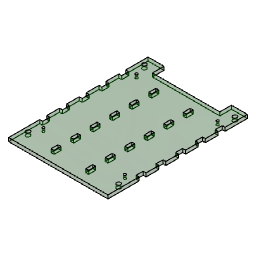
Support_batteries_PCB_KOSMOS3-0 (Autodesk Fusion 360 design; units mm, degrees)
Autodesk Fusion 360 part; units mm, degrees
sketch "Esquisse1" plane through (0, 0, 0) normal (0, 0, 1) x (1, 0, 0)
  line L0 (0, 0) -> (-85.47, 0)
  line L1 (-85.47, 0) -> (-85.47, 120)
  line L2 (0, 120) -> (0, 0)
  circle A0 centre (-81.67, 13) radius 1.75
  circle A1 centre (-3.8, 13) radius 1.75
  circle A2 centre (-81.67, 113) radius 1.75
  circle A3 centre (-3.8, 113) radius 1.75
  line L3 (-71.735, 120) -> (-71.735, 110)
  line L4 (-71.735, 110) -> (-13.735, 110)
  line L5 (-13.735, 110) -> (-13.735, 120)
  line L6 (-85.47, 120) -> (-71.735, 120)
  line L7 (-13.735, 120) -> (0, 120)
  dimension "d1" = 85.47
  dimension "d3" = 77.87
  dimension "d5" = 3.8
  dimension "d6" = 3.5
  dimension "d7" = 3.5
  dimension "d8" = 13
  dimension "d9" = 3.5
  dimension "d10" = 3.5
  dimension "d13" = 13
  dimension "d14" = 3.8
  dimension "d15" = 77.87
  dimension "d16" = 58
  dimension "d17" = 10
  dimension "d18" = 13.735
  dimension "d21" = 120
  dimension "d22" = 7
  dimension "d24" = 7
  constraint horizontal L0
  constraint vertical L1
  constraint vertical L2
  constraint coincident L0.start L2.end
  constraint perpendicular L3 L4
  constraint perpendicular L3 L6
  constraint perpendicular L2 L7
  constraint equal L1 L2
  measures "d1" distance of L0.start L0.end
  measures "d3" distance of A0.centre A1.centre
  measures "d5" distance of L1 A0.centre
  measures "d6" diameter of A1
  measures "d7" diameter of A0
  measures "d8" distance of L0 A0.centre
  measures "d9" diameter of A3
  measures "d10" diameter of A2
  measures "d13" distance of L0 A1.centre
  measures "d14" distance of L1 A2.centre
  measures "d15" distance of A2.centre A3.centre
  measures "d16" distance of L3.end L4.end
  measures "d17" distance of L4.end L5.end
  measures "d18" distance of L2 L5
  measures "d21" distance of L0.start L2.start
  measures "d22" distance of A3.centre L7
  measures "d24" distance of A2.centre L6
extrude "Extrusion1" add sketch "Esquisse1" along normal blind 3
sketch "Esquisse2" plane through (0, 0, 3) normal (0, 0, 1) x (-1, 0, 0)
  circle A0 centre (3.8, -113) radius 1.75
  circle A1 centre (81.67, -113) radius 1.75
  circle A2 centre (3.8, -13) radius 1.75
  circle A3 centre (81.67, -13) radius 1.75
  line L0 (13.735, -120) -> (13.735, -110)
  line L1 (13.735, -110) -> (71.735, -110)
  line L2 (71.735, -110) -> (71.735, -120)
  line L3 (71.735, -120) -> (85.47, -120)
  line L4 (85.47, -120) -> (85.47, 0)
  line L5 (85.47, 0) -> (0, 0)
  line L6 (0, 0) -> (0, -120)
  line L7 (0, -120) -> (13.735, -120)
  line L8 (58.87, -10) -> (56.37, -10)
  line L9 (56.37, -10) -> (56.37, -16)
  line L10 (56.37, -16) -> (58.87, -16)
  line L11 (58.87, -16) -> (58.87, -10)
  line L12 (56.37, -26.8) -> (56.37, -32.8)
  line L13 (56.37, -32.8) -> (58.87, -32.8)
  line L14 (58.87, -26.8) -> (56.37, -26.8)
  line L15 (58.87, -32.8) -> (58.87, -26.8)
  line L16 (56.37, -43.6) -> (56.37, -49.6)
  line L17 (56.37, -49.6) -> (58.87, -49.6)
  line L18 (58.87, -43.6) -> (56.37, -43.6)
  line L19 (58.87, -49.6) -> (58.87, -43.6)
  line L20 (56.37, -60.4) -> (56.37, -66.4)
  line L21 (56.37, -66.4) -> (58.87, -66.4)
  line L22 (58.87, -60.4) -> (56.37, -60.4)
  line L23 (58.87, -66.4) -> (58.87, -60.4)
  line L24 (56.37, -77.2) -> (56.37, -83.2)
  line L25 (56.37, -83.2) -> (58.87, -83.2)
  line L26 (58.87, -77.2) -> (56.37, -77.2)
  line L27 (58.87, -83.2) -> (58.87, -77.2)
  line L28 (56.37, -94) -> (56.37, -100)
  line L29 (56.37, -100) -> (58.87, -100)
  line L30 (58.87, -94) -> (56.37, -94)
  line L31 (58.87, -100) -> (58.87, -94)
  line L32 (42.735, 23.8439) -> (42.735, -200) construction
  line L33 (42.735, 7.0439) -> (42.735, -216.8) construction
  line L34 (29.1, -83.2) -> (26.6, -83.2)
  line L35 (26.6, -10) -> (29.1, -10)
  line L36 (29.1, -16) -> (26.6, -16)
  line L37 (29.1, -66.4) -> (26.6, -66.4)
  line L38 (29.1, -10) -> (29.1, -16)
  line L39 (29.1, -49.6) -> (26.6, -49.6)
  line L40 (26.6, -77.2) -> (29.1, -77.2)
  line L41 (26.6, -94) -> (29.1, -94)
  line L42 (26.6, -49.6) -> (26.6, -43.6)
  line L43 (29.1, -77.2) -> (29.1, -83.2)
  line L44 (29.1, -94) -> (29.1, -100)
  line L45 (26.6, -83.2) -> (26.6, -77.2)
  line L46 (29.1, -32.8) -> (26.6, -32.8)
  line L47 (29.1, -26.8) -> (29.1, -32.8)
  line L48 (29.1, -60.4) -> (29.1, -66.4)
  line L49 (26.6, -26.8) -> (29.1, -26.8)
  line L50 (26.6, -32.8) -> (26.6, -26.8)
  line L51 (26.6, -60.4) -> (29.1, -60.4)
  line L52 (26.6, -16) -> (26.6, -10)
  line L53 (29.1, -43.6) -> (29.1, -49.6)
  line L54 (29.1, -100) -> (26.6, -100)
  line L55 (26.6, -100) -> (26.6, -94)
  line L56 (26.6, -43.6) -> (29.1, -43.6)
  line L57 (26.6, -66.4) -> (26.6, -60.4)
  line L58 (85.47, -26.8) -> (82.97, -26.8)
  line L59 (82.97, -26.8) -> (82.97, -32.8)
  line L60 (82.97, -32.8) -> (85.47, -32.8)
  line L61 (85.47, -32.8) -> (85.47, -26.8)
  line L62 (82.97, -43.8) -> (82.97, -49.8)
  line L63 (82.97, -49.8) -> (85.47, -49.8)
  line L64 (85.47, -49.8) -> (85.47, -43.8)
  line L65 (85.47, -43.8) -> (82.97, -43.8)
  line L66 (82.97, -60.8) -> (82.97, -66.8)
  line L67 (82.97, -66.8) -> (85.47, -66.8)
  line L68 (85.47, -66.8) -> (85.47, -60.8)
  line L69 (85.47, -60.8) -> (82.97, -60.8)
  line L70 (82.97, -77.8) -> (82.97, -83.8)
  line L71 (82.97, -83.8) -> (85.47, -83.8)
  line L72 (85.47, -83.8) -> (85.47, -77.8)
  line L73 (85.47, -77.8) -> (82.97, -77.8)
  line L74 (82.97, -94.8) -> (82.97, -100.8)
  line L75 (82.97, -100.8) -> (85.47, -100.8)
  line L76 (85.47, -100.8) -> (85.47, -94.8)
  line L77 (85.47, -94.8) -> (82.97, -94.8)
  line L78 (2.5, -43.8) -> (2.5, -49.8)
  line L79 (2.5, -100.8) -> (0, -100.8)
  line L80 (0, -49.8) -> (0, -43.8)
  line L81 (2.5, -77.8) -> (2.5, -83.8)
  line L82 (0, -83.8) -> (0, -77.8)
  line L83 (0, -77.8) -> (2.5, -77.8)
  line L84 (0, -26.8) -> (2.5, -26.8)
  line L85 (0, -32.8) -> (0, -26.8)
  line L86 (2.5, -49.8) -> (0, -49.8)
  line L87 (0, -100.8) -> (0, -94.8)
  line L88 (0, -60.8) -> (2.5, -60.8)
  line L89 (2.5, -32.8) -> (0, -32.8)
  line L90 (2.5, -83.8) -> (0, -83.8)
  line L91 (2.5, -94.8) -> (2.5, -100.8)
  line L92 (2.5, -66.8) -> (0, -66.8)
  line L93 (2.5, -26.8) -> (2.5, -32.8)
  line L94 (2.5, -60.8) -> (2.5, -66.8)
  line L95 (0, -43.8) -> (2.5, -43.8)
  line L96 (0, -66.8) -> (0, -60.8)
  line L97 (0, -94.8) -> (2.5, -94.8)
  dimension "d25" = 2.5
  dimension "d26" = 6
  dimension "d27" = 26.6
  dimension "d31" = -20
  dimension "d32" = -84
  dimension "d35" = 85.47
  dimension "d37" = 42.735
  dimension "d42" = 2.5
  dimension "d43" = 6
  dimension "d44" = 26.8
  dimension "d45" = 26.8
  dimension "d48" = 0
  dimension "d49" = -68
  constraint horizontal L8
  constraint vertical L9
  constraint horizontal L10
  constraint vertical L11
  constraint perpendicular L1 L32
  constraint horizontal L58
  constraint vertical L59
  constraint horizontal L60
  constraint vertical L61
  constraint coincident L4 L58.start
  measures "d25" distance of L8.start L8.end
  measures "d26" distance of L8.start L10.end
  measures "d27" distance of L4 L11
  measures "d35" distance of L4.end L5.end
  measures "d37" distance of L4 L32
  measures "d42" distance of L58.start L58.end
  measures "d43" distance of L58.end L59.end
  measures "d44" distance of L5 L14
  measures "d45" distance of L5 L58
extrude "Extrusion2" cut sketch "Esquisse2" against normal blind 3 contours L6 L79 L87 L91 L97 | L6 L81 L82 L83 L90 | L4 L74 L75 L76 L77 | L6 L88 L92 L94 L96 | L4 L70 L71 L72 L73 | L6 L78 L80 L86 L95 | L4 L66 L67 L68 L69 | L6 L84 L85 L89 L93 | L4 L62 L63 L64 L65 | L4 L58 L59 L60 L61 | L8 L9 L10 L11 | L12 L13 L14 L15 | L16 L17 L18 L19 | L20 L21 L22 L23 | L24 L25 L26 L27 | L28 L29 L30 L31 | L34 L40 L43 L45 | L35 L36 L38 L52 | L37 L48 L51 L57 | L39 L42 L53 L56 | L41 L44 L54 L55 | L46 L47 L49 L50
sketch "Esquisse3" plane through (0, 0, 3) normal (0, 0, 1) x (-1, 0, 0)
  line L0 (2.5, -32.8) -> (0, -32.8)
  line L1 (0, -32.8) -> (0, -43.8)
  line L2 (0, -43.8) -> (2.5, -43.8)
  line L3 (2.5, -43.8) -> (2.5, -49.8)
  line L4 (2.5, -49.8) -> (0, -49.8)
  line L5 (0, -49.8) -> (0, -60.8)
  line L6 (0, -60.8) -> (2.5, -60.8)
  line L7 (2.5, -60.8) -> (2.5, -66.8)
  line L8 (2.5, -66.8) -> (0, -66.8)
  line L9 (0, -66.8) -> (0, -77.8)
  line L10 (0, -77.8) -> (2.5, -77.8)
  line L11 (2.5, -77.8) -> (2.5, -83.8)
  line L12 (2.5, -83.8) -> (0, -83.8)
  line L13 (0, -83.8) -> (0, -94.8)
  line L14 (0, -94.8) -> (2.5, -94.8)
  line L15 (2.5, -94.8) -> (2.5, -100.8)
  line L16 (2.5, -100.8) -> (0, -100.8)
  line L17 (0, -100.8) -> (0, -120)
  line L18 (0, -120) -> (13.735, -120)
  line L19 (13.735, -120) -> (13.735, -110)
  line L20 (13.735, -110) -> (71.735, -110)
  line L21 (71.735, -110) -> (71.735, -120)
  line L22 (71.735, -120) -> (85.47, -120)
  line L23 (85.47, -120) -> (85.47, -100.8)
  line L24 (85.47, -100.8) -> (82.97, -100.8)
  line L25 (82.97, -100.8) -> (82.97, -94.8)
  line L26 (82.97, -94.8) -> (85.47, -94.8)
  line L27 (85.47, -94.8) -> (85.47, -83.8)
  line L28 (85.47, -83.8) -> (82.97, -83.8)
  line L29 (82.97, -83.8) -> (82.97, -77.8)
  line L30 (82.97, -77.8) -> (85.47, -77.8)
  line L31 (85.47, -77.8) -> (85.47, -66.8)
  line L32 (85.47, -66.8) -> (82.97, -66.8)
  line L33 (82.97, -66.8) -> (82.97, -60.8)
  line L34 (82.97, -60.8) -> (85.47, -60.8)
  line L35 (85.47, -60.8) -> (85.47, -49.8)
  line L36 (85.47, -49.8) -> (82.97, -49.8)
  line L37 (82.97, -49.8) -> (82.97, -43.8)
  line L38 (82.97, -43.8) -> (85.47, -43.8)
  line L39 (85.47, -43.8) -> (85.47, -32.8)
  line L40 (85.47, -32.8) -> (82.97, -32.8)
  line L41 (82.97, -32.8) -> (82.97, -26.8)
  line L42 (82.97, -26.8) -> (85.47, -26.8)
  line L43 (85.47, -26.8) -> (85.47, 0)
  line L44 (85.47, 0) -> (0, 0)
  line L45 (0, 0) -> (0, -26.8)
  line L46 (0, -26.8) -> (2.5, -26.8)
  line L47 (2.5, -26.8) -> (2.5, -32.8)
  line L48 (56.37, -26.8) -> (58.87, -26.8)
  line L49 (58.87, -26.8) -> (58.87, -32.8)
  line L50 (58.87, -32.8) -> (56.37, -32.8)
  line L51 (56.37, -32.8) -> (56.37, -26.8)
  line L52 (29.1, -26.8) -> (29.1, -32.8)
  line L53 (29.1, -32.8) -> (26.6, -32.8)
  line L54 (26.6, -32.8) -> (26.6, -26.8)
  line L55 (26.6, -26.8) -> (29.1, -26.8)
  line L56 (29.1, -10) -> (29.1, -16)
  line L57 (29.1, -16) -> (26.6, -16)
  line L58 (26.6, -16) -> (26.6, -10)
  line L59 (26.6, -10) -> (29.1, -10)
  line L60 (56.37, -10) -> (58.87, -10)
  line L61 (58.87, -10) -> (58.87, -16)
  line L62 (58.87, -16) -> (56.37, -16)
  line L63 (56.37, -16) -> (56.37, -10)
  line L64 (29.1, -60.4) -> (29.1, -66.4)
  line L65 (29.1, -66.4) -> (26.6, -66.4)
  line L66 (26.6, -66.4) -> (26.6, -60.4)
  line L67 (26.6, -60.4) -> (29.1, -60.4)
  line L68 (29.1, -77.2) -> (29.1, -83.2)
  line L69 (29.1, -83.2) -> (26.6, -83.2)
  line L70 (26.6, -83.2) -> (26.6, -77.2)
  line L71 (26.6, -77.2) -> (29.1, -77.2)
  line L72 (29.1, -94) -> (29.1, -100)
  line L73 (29.1, -100) -> (26.6, -100)
  line L74 (26.6, -100) -> (26.6, -94)
  line L75 (26.6, -94) -> (29.1, -94)
  line L76 (56.37, -60.4) -> (58.87, -60.4)
  line L77 (58.87, -60.4) -> (58.87, -66.4)
  line L78 (58.87, -66.4) -> (56.37, -66.4)
  line L79 (56.37, -66.4) -> (56.37, -60.4)
  line L80 (56.37, -43.6) -> (58.87, -43.6)
  line L81 (58.87, -43.6) -> (58.87, -49.6)
  line L82 (58.87, -49.6) -> (56.37, -49.6)
  line L83 (56.37, -49.6) -> (56.37, -43.6)
  line L84 (29.1, -49.6) -> (26.6, -49.6)
  line L85 (26.6, -49.6) -> (26.6, -43.6)
  line L86 (26.6, -43.6) -> (29.1, -43.6)
  line L87 (29.1, -43.6) -> (29.1, -49.6)
  line L88 (56.37, -94) -> (58.87, -94)
  line L89 (58.87, -94) -> (58.87, -100)
  line L90 (58.87, -100) -> (56.37, -100)
  line L91 (56.37, -100) -> (56.37, -94)
  line L92 (56.37, -77.2) -> (58.87, -77.2)
  line L93 (58.87, -77.2) -> (58.87, -83.2)
  line L94 (58.87, -83.2) -> (56.37, -83.2)
  line L95 (56.37, -83.2) -> (56.37, -77.2)
  circle A0 centre (81.67, -113) radius 1.75
  circle A1 centre (81.67, -13) radius 1.75
  circle A2 centre (3.8, -13) radius 1.75
  circle A3 centre (3.8, -113) radius 1.75
  circle A4 centre (77.97, -102.5) radius 1.05
  circle A5 centre (7.97, -102.5) radius 1.05
  circle A6 centre (77.97, -22.5) radius 1.05
  circle A7 centre (7.97, -22.5) radius 1.05
  dimension "d52" = 2.1
  dimension "d53" = 7.5
  dimension "d54" = 5
  dimension "d57" = -70
  dimension "d58" = 80
  measures "d52" diameter of A4
  measures "d53" distance of L20 A4.centre
  measures "d54" distance of L25 A4.centre
extrude "Extrusion3" cut sketch "Esquisse3" against normal blind 5 contours A4 | A5 | A6 | A7
equation "d18 = ( d1 - d16 ) / 2"
equation "d37 = 85.47 mm / 2"
equation "d42 = d25"
equation "d43 = d26"
